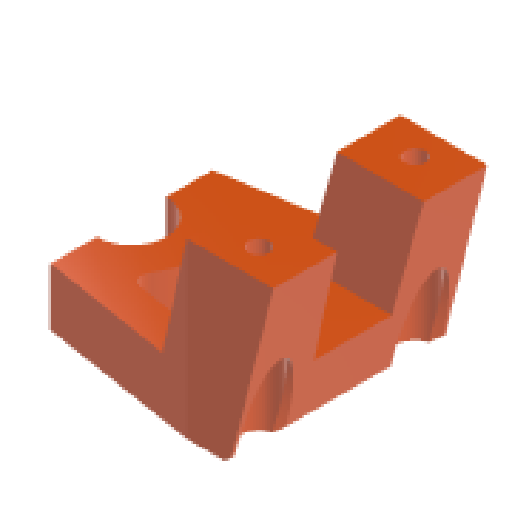
# Autodesk Inventor part: Z Axis Top Brace
Saved by Autodesk Inventor 2023.2 (Build 272271000, 271)
## iProperties
Created: 2023-02-04
Part Number: Z Axis Top Brace
Material: ABS Plastic
Document SubType Name: Modeling
Designer: remop
Density: 1.06 g/cm^3
Appearance: Smooth - Light Orange
Author: remop
Autodesk Inventor part; units mm, degrees
ref_plane "YZ Plane" through (0, 0, 0) normal (1, 0, 0) x (0, 1, 0)
ref_plane "XZ Plane" through (0, 0, 0) normal (0, 1, 0) x (-1, 0, 0)
ref_plane "XY Plane" through (0, 0, 0) normal (0, 0, 1) x (1, 0, 0)
sketch "Sketch1" plane through (0, 0, 0) normal (0, 1, 0) x (-1, 0, 0)
  circle A0 centre (0, 0) radius 6
  line L0 (-28, -18.5) -> (-28, 18.5)
  line L1 (-28, 18.5) -> (0, 14)
  line L2 (0, 14) -> (0, 6)
  line L3 (0, -6) -> (0, -14)
  line L4 (0, -14) -> (-28, -18.5)
  dimension "d0" = 12
  dimension "d1" = 8
  dimension "d2" = 28
  dimension "d9" = 37
  constraints: 10 end point, 2 equal length, 2 point on circle, 2 point on line, 1 centre point, 1 coincident, 1 parallel, 1 vertical, 1 vertical alignment
  measures "d0" diameter of A0
  measures "d1" distance of L1.end L2.end
  measures "d2" distance between parallel lines of L3 L0
  measures "d9" distance of L0.start L0.end
extrude "Extrusion1" add sketch "Sketch1" along normal blind 10 contours A0 L3 L4 L0 L1 L2
sketch "Sketch2" plane through (28, 0, 18.5) normal (1, 0, 0) x (0, 0, -1)
  line L0 (0, 0) -> (37, 0) projected
  line L1 (37, 0) -> (37, 10) projected
  line L2 (0, 10) -> (37, 10) projected
  line L3 (0, 0) -> (0, 10) projected
  line L4 (0, 10) -> (37, 10) projected
  line L5 (0, 10) -> (0, 30)
  line L6 (0, 30) -> (37, 30)
  line L7 (37, 30) -> (37, 10)
  point P0 (18.5, 0)
  dimension "d8" = 20
  constraints: 6 end point, 2 perpendicular, 1 vertical
  measures "d8" distance of L2.start L5.end
extrude "Extrusion2" add sketch "Sketch2" along normal blind 15
chamfer "Chamfer1" distance 5 distance2 20 1 edges at (28, 10, 0) measured on face at (20.6521, 10, 0.2411)
sketch "Sketch3" plane through (0, 10, 0) normal (0, 1, 0) x (1, 0, 0)
  line L0 (23, 17.6964) -> (0, 14) projected
  line L1 (0, 14) -> (0, 6) projected
  arc A0 (0, -6) -> (0, 6) centre (0, 0) ccw projected
  line L2 (0, -6) -> (0, -14) projected
  line L3 (0, -14) -> (23, -17.6964) projected
  circle A1 centre (0, 0) radius 12
  line L4 (7.7432, 9.1675) -> (25.5, 12.0212)
  line L5 (7.7432, -9.1675) -> (28, -12.423)
  line L6 (28, -18.5) -> (28, 18.5) projected
  line L7 (23, 17.6964) -> (23, -17.6964) projected
  point P0 (28, 18.5)
  point P1 (11.5, 15.8482)
  point P2 (23, -11.6194)
  point P3 (23, 11.6194)
  dimension "d10" = 6
  dimension "d11" = 6
  dimension "d12" = 6
  constraints: 4 end point, 2 parallel, 2 point on circle, 1 centre point, 1 coincident, 1 midpoint, 2 other
  measures "d10" radial gap between concentric circles of A1 A0
  measures "d11" distance from line of point (11.5, 15.848) L4
  measures "d12" distance between parallel lines of L3 L5
extrude "Extrusion3" cut sketch "Sketch3" against normal blind 15 contours L7 L5 A1 L4
fillet "Fillet1" radius 2 4 edges at (7.7432, 5, 9.1675) (7.7432, 5, -9.1675) (23, 5, 11.6194) (23, 5, -11.6194)
sketch "Sketch4" plane through (43, 0, -18.5) normal (0, 0, -1) x (-1, 0, 0)
  line L0 (15, 0) -> (43, 0) projected
  line L1 (43, 0) -> (43, 10) projected
  line L2 (20, 10) -> (43, 10) projected
  line L3 (15, 30) -> (20, 10) projected
  line L4 (15, 0) -> (15, 30) projected
  line L5 (15, 0) -> (15, 30) projected
  line L6 (15, 30) -> (0, 30) projected
  line L7 (0, 0) -> (0, 30) projected
  line L8 (15, 0) -> (0, 0) projected
  line L9 (0, 30) -> (0, 0) projected
  line L10 (0, 30) -> (7.5, 0)
  constraints: 2 end point, 1 midpoint, 1 parallel
extrude "Extrusion4" cut sketch "Sketch4" against normal through all contours L8 L7 L10
sketch "Sketch5" plane through (0, 0, 0) normal (0, -1, 0) x (1, 0, 0)
  line L0 (35.5, -18.5) -> (35.5, 18.5) projected
  line L1 (28, 18.5) -> (35.5, 18.5) projected
  line L2 (0, 14) -> (28, 18.5) projected
  line L3 (0, 6) -> (0, 14) projected
  arc A0 (0, -6) -> (0, 6) centre (0, 0) ccw projected
  line L4 (0, -14) -> (0, -6) projected
  line L5 (28, -18.5) -> (0, -14) projected
  line L6 (28, -18.5) -> (35.5, -18.5) projected
  arc A1 (9.9827, -6.6592) -> (9.9827, 6.6592) centre (0, 0) ccw projected
  arc A2 (11.3291, 9.7438) -> (9.9827, 6.6592) centre (11.6465, 7.7691) ccw projected
  line L7 (11.3291, 9.7438) -> (20.6826, 11.247) projected
  line L8 (23, 9.2723) -> (23, -9.2723) projected
  line L9 (20.6826, -11.247) -> (11.3291, -9.7438) projected
  arc A3 (9.9827, -6.6592) -> (11.3291, -9.7438) centre (11.6465, -7.7691) ccw projected
  line L10 (35.5, 18.5) -> (43, 18.5) projected
  line L11 (35.5, -18.5) -> (35.5, 18.5) projected
  line L12 (43, -18.5) -> (35.5, -18.5) projected
  line L13 (43, -18.5) -> (43, 18.5) projected
  line L14 (35.5, -18.5) -> (35.5, 18.5) projected
  arc A4 (23, 9.2723) -> (20.6826, 11.247) centre (21, 9.2723) ccw projected
  arc A5 (20.6826, -11.247) -> (23, -9.2723) centre (21, -9.2723) ccw projected
  point P0 (35.5, 13.5)
  point P1 (35.5, -13.5)
  point P2 (39.25, 18.5)
  dimension "d21" = 5
  dimension "d22" = 5
  constraints: 2 point on line, 1 midpoint
  measures "d21" distance from line of L12 point (35.5, -13.5)
  measures "d22" vertical distance of point (39.25, 18.5) point (35.5, 13.5)
hole "Hole1" at (35.5, 0, 13.5) at (35.5, 0, -13.5) direction (0, 1, 0) diameter 3.6 end through all counterbore diameter 7 counterbore depth 26 clearance for "Hex Head Cap Screw ISO 24017" size "M3" standard "ISO"
chamfer "Chamfer2" distance 1 angle 45 5 edges at (39, 14, 13.5) (39, 14, -13.5) (35.5, 0, 0) (35.5, 0, -17.75) (35.5, 0, 17.75)
sketch "Sketch7" plane through (0, 0, -14) normal (-1, 0, 0) x (0, 0, 1)
  line L0 (-4.5, 30) -> (-3.6964, 10) projected
  line L1 (23.2723, 10) -> (31.6964, 10) projected
  line L2 (4.7277, 10) -> (23.2723, 10) projected
  line L3 (-3.6964, 10) -> (4.7277, 10) projected
  line L4 (32.5, 30) -> (31.6964, 10) projected
  line L5 (-4.5, 30) -> (32.5, 30) projected
  line L6 (-4.5, 30) -> (32.5, 30) projected
  line L7 (6.5089, 30) -> (7.2723, 11)
  line L8 (7.2723, 11) -> (20.7277, 11)
  line L9 (20.7277, 11) -> (21.4911, 30)
  point P0 (14, 0)
  dimension "d33" = 11
  dimension "d34" = 11
  dimension "d35" = 1
  constraints: 6 end point, 3 parallel, 2 horizontal alignment, 2 point on line
  measures "d33" distance between parallel lines of L0 L7
  measures "d34" distance between parallel lines of L4 L9
  measures "d35" distance between parallel lines of L2 L8
extrude "Extrusion5" cut sketch "Sketch7" against normal through all contours L5 L9 L8 L7
sketch "Sketch8" plane through (0, 0, -14) normal (-1, 0, 0) x (0, 0, 1)
  line L0 (0, 0) -> (8, 0) projected
  line L1 (8, 0) -> (8, 10) projected
  line L2 (0, 10) -> (8, 10) projected
  line L3 (0, 0) -> (0, 10) projected
  line L4 (20, 0) -> (28, 0) projected
  line L5 (28, 0) -> (28, 10) projected
  line L6 (20, 10) -> (28, 10) projected
  line L7 (20, 0) -> (20, 10) projected
  point P0 (14, 0)
  point P1 (4, 5)
  point P2 (24, 5)
  point P3 (4, 10)
  point P4 (24, 10)
  point P5 (8, 5)
  point P6 (20, 5)
  constraints: 4 midpoint, 2 horizontal alignment, 2 vertical alignment
hole "Hole2" at (0, 5, -10) at (0, 5, 10) direction (1, 0, 0) diameter 2.8 depth 8 tip angle 118
equation "\"d11\" = d10"
equation "\"d12\" = d10"
equation "\"d22\" = d21"
equation "\"d34\" = d33"
body "Solid1"
